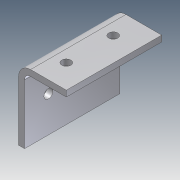
# Autodesk Inventor part: GE-12061
Saved by Autodesk Inventor 2012 (Build 160160000, 160)
## iProperties
Created: 2011-11-08
Part Number: GE-12061
Document SubType Name: Modeling
Designer: dfoster
Density: 1 g/cm^3
Description: Bridge Sensor Bracket
Material: Default
Title: Bridge Sensor Bracket
Author: dfoster
Autodesk Inventor part; units mm, degrees
ref_plane "YZ Plane" through (0, 0, 0) normal (1, 0, 0) x (0, 1, 0)
ref_plane "XZ Plane" through (0, 0, 0) normal (0, 1, 0) x (-1, 0, 0)
ref_plane "XY Plane" through (0, 0, 0) normal (0, 0, 1) x (1, 0, 0)
sketch "Sketch1" plane through (0, 0, 0) normal (0, 0, 1) x (1, 0, 0)
  line L0 (6.35, 0) -> (25.4, 0)
  line L1 (25.4, 0) -> (25.4, -3.175)
  line L2 (25.4, -3.175) -> (6.35, -3.175)
  line L3 (3.175, -6.35) -> (3.175, -38.1)
  line L4 (3.175, -38.1) -> (0, -38.1)
  line L5 (0, -38.1) -> (0, -6.35)
  arc A0 (6.35, -3.175) -> (3.175, -6.35) centre (6.35, -6.35) ccw
  arc A1 (6.35, 0) -> (0, -6.35) centre (6.35, -6.35) ccw
  point P0 (0, 0)
  dimension "d0" = 3.175
  dimension "d1" = 38.1
  dimension "d2" = 3.175
  dimension "d3" = 6.35
  dimension "d6" = 25.4
  constraints: 12 end point, 4 parallel, 4 point on circle, 4 tangent, 2 centre point, 2 perpendicular, 2 point on line, 1 horizontal
  measures "d0" distance of L3.end L4.end
  measures "d1" distance of L4.end point (0, 0)
  measures "d2" radius of A0
  measures "d3" radius of A1
  measures "d6" distance between parallel lines of L5 L1
extrude "Extrusion1" add sketch "Sketch1" along normal blind 50.8
hole "Hole1" at (12.7, -3.175, 38.1) direction (0, 1, 0) diameter 4.826 depth 25.4 tip angle 118
pattern_linear "Rectangular Pattern1" count 2 spacing 25 along (0, 0, -1) of "Hole1"
hole "Hole2" at (3.175, -19.05, 38.1) direction (-1, 0, 0) diameter 4.826 depth 25.4 tip angle 118
pattern_linear "Rectangular Pattern2" count 2 spacing 25.4 along (0, 0, -1) of "Hole2"
body "Solid1"
